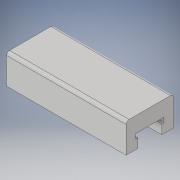
# Autodesk Inventor part: rail holder
Saved by Autodesk Inventor 2019 (Build 230136000, 136)
## iProperties
Created: 2018-11-20
Part Number: rail holder
Material: Generic
Document SubType Name: Modeling
Designer: jprado
Density: 1 g/cm^3
Appearance: Default
Author: jprado
Autodesk Inventor part; units mm, degrees
ref_plane "YZ Plane" through (0, 0, 0) normal (1, 0, 0) x (0, 1, 0)
ref_plane "XZ Plane" through (0, 0, 0) normal (0, 1, 0) x (-1, 0, 0)
ref_plane "XY Plane" through (0, 0, 0) normal (0, 0, 1) x (1, 0, 0)
sketch "Sketch1" plane through (0, 0, 0) normal (0, 1, 0) x (-1, 0, 0)
  line L0 (81, 0) -> (0, 0)
  line L1 (0, 0) -> (0, -32)
  line L2 (0, -32) -> (81, -32)
  line L3 (81, -32) -> (81, 0)
  point P0 (0, -16)
  point P1 (40.5, 0)
  dimension "d0" = 81
  dimension "d1" = 32
  constraints: 8 end point, 2 midpoint, 2 parallel, 1 horizontal, 1 horizontal alignment, 1 perpendicular, 1 vertical alignment
  measures "d0" distance of L0.start L0.end
  measures "d1" distance of L2.end L0.start
extrude "Extrusion1" add sketch "Sketch1" along normal blind 20
sketch "Sketch2" plane through (0, 0, 0) normal (1, 0, 0) x (0, 0, -1)
  line L0 (0, 0) -> (32, 0) projected
  line L1 (24.1, 0) -> (24.1, 6.35)
  line L2 (24.1, 6.35) -> (25.6, 6.35)
  line L3 (25.6, 6.35) -> (25.6, 9.525)
  line L4 (25.6, 9.525) -> (6.4, 9.525)
  line L5 (6.4, 9.525) -> (6.4, 6.35)
  line L6 (6.4, 6.35) -> (7.9, 6.35)
  line L7 (7.9, 6.35) -> (7.9, 0)
  line L8 (24.1, 0) -> (7.9, 0)
  line L9 (32, 0) -> (32, 20) projected
  line L10 (0, 0) -> (0, 20) projected
  dimension "d4" = 3.175
  dimension "d5" = 6.35
  dimension "d6" = 19.2
  dimension "d7" = 16.2
  dimension "d8" = 6.4
  dimension "d17" = 7.9
  dimension "d18" = 32
  constraints: 16 end point, 5 perpendicular, 4 point on line, 1 collinear, 1 vertical
  measures "d4" distance of L2.end L3.end
  measures "d5" distance of L6.end L7.end
  measures "d6" distance of L3.end L4.end
  measures "d7" distance between parallel lines of L7 L1
  measures "d8" distance between parallel lines of L9 L3
  measures "d17" distance between parallel lines of L9 L1
  measures "d18" distance between parallel lines of L9 L10
extrude "Extrusion2" cut sketch "Sketch2" against normal blind 103.1875
fillet "Fillet1" radius 2 1 edges at (-40.5, 20, -32)
fillet "Fillet2" radius 2 1 edges at (-40.5, 20, 0)
equation "\"d8\" = -0.5 * d6 + 0.5 * d18"
equation "\"d17\" = -0.5 * d7 + 0.5 * d18"
body "Solid1"
